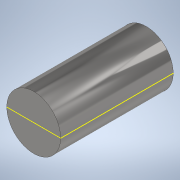
# Autodesk Inventor part: Палец
Saved by Autodesk Inventor 2021 (Build 250183000, 183)
## iProperties
Created: 2020-11-30
Part Number: Палец
Material: Сталь, высокопрочная, низколегированная
Document SubType Name: Modeling
Designer: Тимоха
Mass: 14180.4 g
Surface Area: 879.646 cm^2
Volume: 1806.42 cm^3
Density: 7.85 g/cm^3
Appearance: Сталь — полированная
Author: Тимоха
Autodesk Inventor part; units mm, degrees
ref_plane "YZ Plane" through (0, 0, 0) normal (1, 0, 0) x (0, 1, 0)
ref_plane "XZ Plane" through (0, 0, 0) normal (0, 1, 0) x (-1, 0, 0)
ref_plane "XY Plane" through (0, 0, 0) normal (0, 0, 1) x (1, 0, 0)
sketch "Эскиз1" plane through (0, 0, 0) normal (0, 0, 1) x (1, 0, 0)
  circle A0 centre (0, 0) radius 55
  dimension "d0" = 110
  constraints: 1 centre point, 1 coincident
  measures "d0" diameter of A0
extrude "Выдавливание1" add sketch "Эскиз1" along normal blind 230
sketch "Эскиз2" plane through (0, 0, 0) normal (0, 1, 0) x (-1, 0, 0)
  line L0 (55, 0) -> (-55, 0) projected
  line L1 (-55, 0) -> (-55, 230) projected
  line L2 (55, 230) -> (-55, 230) projected
  line L3 (-55, 230) -> (-55, 222.5)
  line L4 (-55, 222.5) -> (-52, 222.5)
  line L5 (-52, 222.5) -> (-52, 226)
  line L6 (-52, 226) -> (-55, 226)
  line L7 (0, -46) -> (0, 276) projected
  line L8 (-55, 0) -> (-55, 7.5)
  line L9 (-55, 0) -> (-55, 230) projected
  line L10 (-55, 7.5) -> (-52, 7.5)
  line L11 (-52, 7.5) -> (-52, 4)
  line L12 (-52, 4) -> (-55, 4)
  line L13 (-55, 0) -> (-55, 230) projected
  point P0 (0, 0)
  dimension "d3" = 7.5
  dimension "d5" = 7.5
  dimension "d6" = 3.5
  constraints: 16 end point, 6 perpendicular, 4 point on line
  measures "d3" distance of L1.end L3.end
  measures "d5" distance of L1.start L8.end
  measures "d6" distance of L10.end L11.end
revolve "Вращение1" cut sketch "Эскиз2" angle 360 about axis through (0, 0, -10) along (0, 0, 1) contours L1 L10 L11 L12 | L6 L5 L4 L1
